3.1” oled case v17 (Autodesk Fusion 360 design; units mm, degrees)
Autodesk Fusion 360 part; units mm, degrees
note: some values were not read from the file. Chosen so that the rebuilt part matches the saved one: which bodies a step acts on; which face or edge a step refers to. Set by a fixed rule: which sketch regions a step uses.
sketch "onderplaat_display" plane through (0, 0, 0) normal (0, 1, 0) x (1, 0, 0) in component "display"
  line L0 (-50, 20.05) -> (50.3, 20.05)
  line L1 (50.3, 20.05) -> (50.3, -18.05)
  line L2 (50.3, -18.05) -> (-50, -18.05)
  line L3 (-50, -18.05) -> (-50, 20.05)
  circle A0 centre (-47.5, -15.55) radius 1.3
  circle A1 centre (-47.5, 17.55) radius 1.3
  circle A2 centre (47.8, 17.55) radius 1.3
  circle A3 centre (47.8, -15.55) radius 1.3
  line L4 (45, 14.7) -> (-45, 14.7)
  line L5 (-45, 14.7) -> (-45, -14.7)
  line L6 (-45, -14.7) -> (45, -14.7)
  line L7 (45, -14.7) -> (45, 14.7)
  line L8 (0, -14.7) -> (0, 14.7) construction
  line L9 (-45, 0) -> (45, 0) construction
  line L10 (0, -14.7) -> (32.13, -14.7)
  line L11 (32.13, -14.7) -> (32.13, -17.2)
  line L12 (0, -14.7) -> (-31.87, -14.7)
  line L13 (-31.87, -14.7) -> (-31.87, -17.2)
  line L14 (-31.87, -17.2) -> (32.13, -17.2)
  line L15 (-39.1, 10.35) -> (39.1, 10.35)
  line L16 (39.1, 10.35) -> (39.1, -10.35)
  line L17 (39.1, -10.35) -> (-39.1, -10.35)
  line L18 (-39.1, -10.35) -> (-39.1, 10.35)
  line L19 (-39.1, 0) -> (39.1, 0) construction
  line L20 (0, -10.35) -> (0, 0) construction
  line L21 (0, -14.7) -> (0, 0)
  dimension "d2" = 100.3
  dimension "d3" = 38.1
  dimension "d9" = 2.6
  dimension "d10" = 2.5
  dimension "d11" = 2.5
  dimension "d12" = 2.5
  dimension "d13" = 2.5
  dimension "d14" = 2.5
  dimension "d15" = 2.5
  dimension "d16" = 2.5
  dimension "d17" = 2.5
  dimension "d18" = 29.4
  dimension "d19" = 2.85
  dimension "d20" = 50
  dimension "d25" = 18.13
  dimension "d26" = 64
  dimension "d27" = 2.5
  dimension "d28" = 5
  dimension "d36" = 20.7
  dimension "d37" = 78.2
  measures "d2" distance of L0.start L0.end
  measures "d3" distance of L0.end L1.end
  measures "d9" diameter of A0
  measures "d10" distance of L3 A0.centre
  measures "d11" distance of L2 A0.centre
  measures "d12" distance of L0 A1.centre
  measures "d13" distance of L3 A1.centre
  measures "d14" distance of L1 A2.centre
  measures "d15" distance of L0 A2.centre
  measures "d16" distance of L1 A3.centre
  measures "d17" distance of L2 A3.centre
  measures "d18" distance of L4.start L6.end
  measures "d19" distance of A2.centre L4
  measures "d20" distance of L3 L8
  measures "d25" distance of L3 L13
  measures "d26" distance of L11.end L13.end
  measures "d27" distance of L10.end L11.end
  measures "d28" distance of L3 L5
  measures "d36" distance of L15.end L16.end
  measures "d37" distance of L16.end L17.end
extrude "Extrude1" add sketch "onderplaat_display" along normal blind 1.6 contours L0 L1 L2 L3 makes body 1 in component "display"
extrude "Extrude2" add sketch "onderplaat_display" along normal blind 4.9 contours L4 L5 L6 L7 L10 L12 | L6 L10 L11 L12 L13 L14 | L15 L16 L17 L18 bodies 1 in component "display"
extrude "Extrude3" add sketch "onderplaat_display" against normal blind 2.1 contours L4 L5 L6 L7 L10 L12 | L15 L16 L17 L18 bodies 1 in component "display"
fillet "Fillet1" radius 0.3 8 edges at (-31.87, 4.9, 15.95) (0.13, 4.9, 17.2) (-38.435, 4.9, 14.7) (-45, 4.9, 0) (0, 4.9, -14.7) (45, 4.9, 0) (38.565, 4.9, 14.7) (32.13, 4.9, 15.95) on bodies 1 in component "display"
extrude "Extrude4" cut sketch "onderplaat_display" along normal up to surface (4.9 mm away) contours L15 L16 L17 L18 bodies 1 in component "display"
extrude "Extrude5" add sketch "onderplaat_display" along normal blind 4.4 contours L15 L16 L17 L18 bodies 1 in component "display"
copy_body "CutPasteBodies1" bodies 1 removing the originals makes body 2 in component "display"
sketch "Sketch1" plane through (0, 0, 0) normal (0, 1, 0) x (1, 0, 0) in component "led"
  line L0 (-2.5, 1) -> (2.5, 1)
  line L1 (2.5, 1) -> (2.5, -1)
  line L2 (2.5, -1) -> (-2.5, -1)
  line L3 (-2.5, -1) -> (-2.5, 1)
  line L4 (0, 0) -> (0, 1) construction
  line L5 (0, 0) -> (2.5, 0) construction
  line L6 (-2.5, -1) -> (2.5, -1)
  line L7 (2.5, -1) -> (2.5, -1.3)
  line L8 (2.5, -1.3) -> (-2.5, -1.3)
  line L9 (-2.5, -1.3) -> (-2.5, -1)
  line L10 (-2.5, 1) -> (2.5, 1)
  line L11 (2.5, 1) -> (2.5, 1.3)
  line L12 (2.5, 1.3) -> (-2.5, 1.3)
  line L13 (-2.5, 1.3) -> (-2.5, 1)
  dimension "d117" = 2
  dimension "d118" = 5
  dimension "d121" = 0.3
  dimension "d122" = 0.3
  measures "d117" distance of L0.start L2.end
  measures "d118" distance of L0.start L0.end
  measures "d121" distance of L2.end L8.end
  measures "d122" distance of L0.start L12.end
extrude "Extrude2'" add sketch "Sketch1" along normal blind 7 separate body contours L0 L1 L2 L3 L6 L10 makes body 3 in component "led"
extrude "Extrude3'" add sketch "Sketch1" along normal blind 0.9 contours L0 L10 L11 L12 L13 | L2 L6 L7 L8 L9 bodies 3 in component "led"
chamfer "Chamfer1" distance 0.2 angle 45 1 edges at (0, 0.9, -1.3) on bodies 3 in component "led"
chamfer "Chamfer2" distance 0.2 angle 45 1 edges at (0, 0.9, 1.3) on bodies 3 in component "led"
sketch "Sketch2" plane through (0, 0, 0) normal (0, 0, 1) x (1, 0, 0) in component "led"
  line L0 (-2.5, 0) -> (2.5, 0)
  line L1 (0, 0) -> (0, 3.7069) construction
  line L2 (0, 3.7069) -> (-2, 3.7069)
  line L3 (-2, 3.7069) -> (-2, 1.9116)
  line L4 (-2, 1.9116) -> (0, 1.9116)
  line L5 (0, 1.9116) -> (0, 3.7069)
  line L6 (0, 1.9116) -> (0.7, 2.8)
  line L7 (0.7, 2.8) -> (0.7, 3.6944)
  line L8 (0.7, 3.6944) -> (0, 3.7069)
  line L9 (0.9102, 2.7928) -> (0.9262, 3.6944)
  line L10 (0.9262, 3.6944) -> (2, 3.6944)
  line L11 (2, 3.6944) -> (2, 1.8715)
  line L12 (2, 1.8715) -> (0.4, 1.9)
  line L13 (0.9102, 2.7928) -> (0.4, 1.9)
  line L14 (0.4, 1.9) -> (0, 1.9)
  line L15 (-2, 1.9116) -> (-1.5, 1.9116)
  line L16 (-1.5, 1.9116) -> (-1.5, -1.2931)
  line L17 (-1.5, -1.2931) -> (-2, -1.2931)
  line L18 (-2, -1.2931) -> (-2, 1.9116)
  line L19 (2, 1.8715) -> (1.5, 1.8715)
  line L20 (1.5, 1.8715) -> (1.5, -1.3056)
  line L21 (1.5, -1.3056) -> (2, -1.3056)
  line L22 (2, -1.3056) -> (2, 1.8715)
  line L23 (0.7, 3.6944) -> (2, 3.6944) construction
  point P0 (2.5, 0)
  point P1 (-2.5, 0)
  dimension "d127" = 0.5
  dimension "d128" = 0.5
  dimension "d129" = 0.5
  dimension "d130" = 5
  dimension "d131" = 5
  measures "d127" distance of L22 P0
  measures "d128" distance of L18 P1
  measures "d129" distance of L16.end L17.end
  measures "d130" distance of L2 L17
  measures "d131" distance of L10 L21
extrude "Extrude4'" cut sketch "Sketch2" along normal blind 0.2 and the other way blind 0.2 bodies 3 in component "led"
extrude "Extrude5'" add sketch "Sketch2" along normal blind 0.19 and the other way blind 0.19 separate body makes body 5 at (-1.1667, 3.1084, 0.19) makes body 4 at (1.6367, 2.7862, 0.19) makes body 4 at (1.8333, 0.8125, 0.19) in component "led"
copy_body "CopyPasteBodies1" bodies 4 5 3 makes body 6 makes body 7 makes body 8
move_body "Move1" bodies 6 7 8 to x (1, 0, 0) y (0, 1, 0) z (0, 0, 1) at (-12, -2.4, 19.875)
copy_body "CopyPasteBodies2" bodies 4 5 3 makes body 9 makes body 10 makes body 11
move_body "Move2" bodies 9 10 11 to x (1, 0, 0) y (0, 1, 0) z (0, 0, 1) at (-6, -2.4, 19.875)
copy_body "CopyPasteBodies3" bodies 4 5 3 makes body 12 makes body 13 makes body 14
move_body "Move3" bodies 12 13 14 to x (1, 0, 0) y (0, 1, 0) z (0, 0, 1) at (0, -2.4, 19.875)
copy_body "CopyPasteBodies4" bodies 4 5 3 makes body 15 makes body 16 makes body 17
move_body "Move4" bodies 15 16 17 to x (1, 0, 0) y (0, 1, 0) z (0, 0, 1) at (6, -2.4, 19.875)
copy_body "CopyPasteBodies5" bodies 4 5 3 makes body 18 makes body 19 makes body 20
move_body "Move5" bodies 18 19 20 to x (1, 0, 0) y (0, 1, 0) z (0, 0, 1) at (12, -2.4, 19.875)
sketch "Sketch1 (2)" plane through (0, 1.6, 0) normal (0, 1, 0) x (-1, 0, 0) in component "nice case"
  circle A0 centre (-47.8, -17.55) radius 1.3
  line L0 (-45, 14.7) -> (-32.13, 14.7)
  line L1 (-32.13, 14.7) -> (-32.13, 17.2)
  line L2 (-32.13, 17.2) -> (31.87, 17.2)
  line L3 (31.87, 17.2) -> (31.87, 14.7)
  line L4 (31.87, 14.7) -> (45, 14.7)
  line L5 (45, 14.7) -> (45, -14.7)
  line L6 (45, -14.7) -> (-45, -14.7)
  line L7 (-45, -14.7) -> (-45, 14.7)
  circle A1 centre (-47.8, 15.55) radius 1.3
  circle A2 centre (47.5, 15.55) radius 1.3
  circle A3 centre (47.5, -17.55) radius 1.3
  line L8 (-50.3, 18.05) -> (-50.3, -20.05)
  line L9 (-50.3, -20.05) -> (50, -20.05)
  line L10 (50, -20.05) -> (50, 18.05)
  line L11 (50.35, -20.05) -> (-50.35, -20.05)
  line L12 (-14.5, 21.375) -> (14.5, 21.375)
  line L13 (14.5, 21.375) -> (14.5, 19.375)
  line L14 (14.5, 19.375) -> (-14.5, 19.375)
  line L15 (-14.5, 19.375) -> (-14.5, 21.375)
  line L16 (-3.5, 21.375) -> (-2.5, 21.375)
  line L17 (-2.5, 21.375) -> (-2.5, 19.375)
  line L18 (-2.5, 19.375) -> (-3.5, 19.375)
  line L19 (-3.5, 19.375) -> (-3.5, 21.375)
  line L20 (2.5, 21.375) -> (3.5, 21.375)
  line L21 (3.5, 21.375) -> (3.5, 19.375)
  line L22 (3.5, 19.375) -> (2.5, 19.375)
  line L23 (2.5, 19.375) -> (2.5, 21.375)
  line L24 (8.5, 21.375) -> (9.5, 21.375)
  line L25 (9.5, 21.375) -> (9.5, 19.375)
  line L26 (9.5, 19.375) -> (8.5, 19.375)
  line L27 (8.5, 19.375) -> (8.5, 21.375)
  line L28 (-9.5, 21.375) -> (-8.5, 21.375)
  line L29 (-8.5, 21.375) -> (-8.5, 19.375)
  line L30 (-8.5, 19.375) -> (-9.5, 19.375)
  line L31 (-9.5, 19.375) -> (-9.5, 21.375)
  line L32 (0, 21.375) -> (0, 19.375) construction
  line L33 (-14.5, 21.375) -> (-14.5, 22.55)
  line L34 (14.5, 21.375) -> (14.5, 22.55) construction
  line L35 (-50.35, 18.05) -> (-15.5, 22.55)
  line L36 (15.5, 22.55) -> (50.35, 18.05)
  line L37 (-15.5, 22.55) -> (15.5, 22.55)
  line L38 (-50.35, 18.05) -> (-50.35, -20.05)
  line L39 (50.35, 18.05) -> (50.35, -20.05)
  line L40 (-15.5643, 23.55) -> (15.5643, 23.55)
  line L41 (15.5643, 23.55) -> (51.35, 18.9292)
  line L42 (51.35, 18.9292) -> (51.35, -21.05)
  line L43 (51.35, -21.05) -> (-51.35, -21.05)
  line L44 (-51.35, 18.9292) -> (-51.35, -21.05)
  line L45 (-51.35, 18.9292) -> (-15.5643, 23.55)
  line L46 (15.5, 22.55) -> (-15.5, 22.55)
  line L47 (-15.5, 22.55) -> (-15.5, 18.375)
  line L48 (-15.5, 18.375) -> (15.5, 18.375)
  line L49 (15.5, 18.375) -> (15.5, 22.55)
  line L50 (14.5, -20.05) -> (-14.5, -20.05)
  line L51 (-14.5, -20.05) -> (-14.5, -15.7)
  line L52 (-14.5, -15.7) -> (14.5, -15.7)
  line L53 (14.5, -15.7) -> (14.5, -20.05)
  point P0 (-15.5, 22.55)
  point P1 (15.5, 22.55)
  point P2 (-50.35, 18.05)
  point P3 (50.35, 18.05)
  dimension "d148" = 5.35
  dimension "d160" = 1
  dimension "d161" = 5
  dimension "d162" = 1
  dimension "d163" = 5
  dimension "d164" = 1
  dimension "d165" = 5
  dimension "d166" = 2
  dimension "d167" = 5
  dimension "d168" = 1
  dimension "d169" = 5
  dimension "d172" = 14.5
  dimension "d173" = 1
  dimension "d174" = 1
  dimension "d178" = 5.35
  dimension "d179" = 5.35
  dimension "d180" = 5.35
  dimension "d181" = 1
  dimension "d197" = 29
  dimension "d199" = 14.5
  dimension "d200" = 1
  dimension "d203" = 1.175
  dimension "d204" = 1
  measures "d148" distance of L6 L11
  measures "d160" distance of L17 L19
  measures "d161" distance of L17 L23
  measures "d162" distance of L21 L23
  measures "d163" distance of L21 L27
  measures "d164" distance of L25 L27
  measures "d165" distance of L13 L25
  measures "d166" distance of L12.start L14.end
  measures "d167" distance of L15 L31
  measures "d168" distance of L29 L31
  measures "d169" distance of L19 L29
  measures "d172" distance of L13 origin
  measures "d173" distance of L33.end P0
  measures "d174" distance of L34.end P1
  measures "d178" distance of L7 L38
  measures "d179" distance of L2 L37
  measures "d180" distance of L5 L39
  measures "d197" distance of L50.start L50.end
  measures "d199" distance of origin L53
  measures "d200" distance of L6 L52
  measures "d203" distance of L12 L37
  measures "d204" distance of L14 L48
extrude "Extrude1'" add sketch "Sketch1 (2)" along normal blind 3 separate body contours A0 | A1 | A2 | A3 | L9 L11 L35 L36 L38 L39 L47 L48 L49 L51 L52 L53 | L9 L11 L50 L51 L52 L53 | L37 L46 L47 L48 L49 | L12 L14 L28 L29 L30 L31 | L12 L14 L16 L17 L18 L19 | L12 L14 L20 L21 L22 L23 | L12 L14 L24 L25 L26 L27 | L40 L41 L42 L43 L44 L45 makes body 21 in component "nice case"
extrude "Extrude2''" add sketch "Sketch1 (2)" against normal blind 6 contours L40 L41 L42 L43 L44 L45 bodies 21 in component "nice case"
extrude "Extrude3''" add sketch "Sketch1 (2)" against normal blind 1.6 draft -10 contours A0 | A1 | A2 | A3 bodies 21 in component "nice case"
extrude "Extrude4''" add sketch "Sketch1 (2)" against normal blind 3.3 contours L37 L46 L47 L48 L49 | L12 L14 L28 L29 L30 L31 | L12 L14 L16 L17 L18 L19 | L12 L14 L20 L21 L22 L23 | L12 L14 L24 L25 L26 L27 bodies 21 in component "nice case"
fillet "Fillet3" radius 1 2 edges at (15.5, -0.05, 22.55) (-15.5, -0.05, 22.55) on bodies 21 in component "nice case"
fillet "Fillet4" radius 1 7 edges at (51.35, 0.1, 18.9292) (33.4571, 4.6, 21.2396) (51.35, 4.6, -1.0604) (0, 4.6, 23.55) (-33.4571, 4.6, 21.2396) (-51.35, 4.6, -1.0604) (-51.35, 0.1, 18.9292) on bodies 21 in component "nice case"
extrude "Extrude5''" cut sketch "Sketch1 (2)" along normal blind 2 contours L9 L11 L50 L51 L52 L53 bodies 21 in component "nice case"
move_body "Move6" bodies 18 19 20 15 17 16 to x (1, 0, 0) y (0, 1, 0) z (0, 0, 1) at (0, 0, 0.5)
move_body "Move7" bodies 7 6 10 9 13 12 14 11 8 to x (1, 0, 0) y (0, 1, 0) z (0, 0, 1) at (0, 0, 0.5)
fillet "Fillet5" radius 1 5 edges at (51.35, -0.4, -21.05) (51.0571, 4.3071, -21.05) (0, 4.6, -21.05) (-51.0571, 4.3071, -21.05) (-51.35, -0.4, -21.05) on bodies 21 in component "nice case"
component "display" placed x (1, 0, 0) y (0, 1, 0) z (0, 0, 1) at (0, 0, 0)
component "led" placed x (1, 0, 0) y (0, 1, 0) z (0, 0, 1) at (0, 0, 0)
component "nice case" placed x (1, 0, 0) y (0, 1, 0) z (0, 0, 1) at (0, 0, 0)
named bodies: "display", "display_body", "glas", "pootje1", "pootje2", "pootje1 (1)", "pootje2 (1)", "glas (1)", "pootje1 (2)", "pootje2 (2)", "glas (2)", "pootje1 (3)", "pootje2 (3)", "glas (3)", "pootje1 (4)", "pootje2 (4)", "glas (4)"
